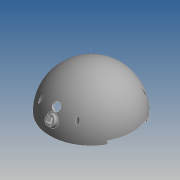
# Autodesk Inventor part: I000
Saved by Autodesk Inventor 2017 (Build 210142000, 142)
## iProperties
Created: 2018-10-05
Part Number: I000
Material: ABS
Document SubType Name: Modeling
Designer: Gilles Mottiez
Density: 1.06 g/cm^3
Appearance: Par défaut
Description: Demi-coque arrière
Mass: 97.4809 g
Surface Area: 629.597 cm^2
Volume: 91.9632 cm^3
Author: Gilles Mottiez
Autodesk Inventor part; units mm, degrees
ref_plane "YZ Plane" through (0, 0, 0) normal (1, 0, 0) x (0, 1, 0)
ref_plane "XZ Plane" through (0, 0, 0) normal (0, 1, 0) x (-1, 0, 0)
sketch "Sketch1" plane through (0, 0, 0) normal (0, 0, 1) x (1, 0, 0)
  circle A0 centre (0, 0) radius 70 construction
  line L0 (-70, 0) -> (70, 0) construction
  arc A1 (70, 0) -> (-70, 0) centre (0, 0) ccw
  line L1 (-70, 0) -> (70, 0)
  dimension "d0" = 140
  constraints: 4 end point, 4 point on circle, 2 centre point, 2 coincident, 1 collinear, 1 concentric, 1 horizontal, 1 midpoint
  measures "d0" diameter of A0
revolve "Révolution1" add sketch "Sketch1" angle 180 about axis through (-70, 0, 0) along (1, 0, 0)
sketch "Esquisse2" plane through (0, 0, 0) normal (1, 0, 0) x (0, 1, 0)
  line L0 (-70, 0) -> (70, 0) construction
  circle A0 centre (0, 0) radius 67 construction
  arc A1 (67, 0) -> (-67, 0) centre (0, 0) ccw
  line L1 (67, 0) -> (-67, 0)
  dimension "d2" = 134
  constraints: 4 point on circle, 2 centre point, 2 concentric, 2 end point, 2 point on line, 1 coincident, 1 collinear
  measures "d2" diameter of A0
revolve "Révolution2" cut sketch "Esquisse2" angle 360 about axis through (0, 67, 0) along (0, -1, 0)
sketch "Esquisse3" plane through (0, 0, 0) normal (1, 0, 0) x (0, 1, 0)
  line L0 (67, 0) -> (-67, 0) construction
  line L1 (-70, 0) -> (70, 0) construction
  arc A0 (70, 0) -> (-70, 0) centre (0, 0) ccw construction
  line L2 (32.5, 0) -> (-32.5, 0)
  line L3 (-32.5, 0) -> (-32.5, 5.5)
  line L4 (-32.5, 5.5) -> (32.5, 5.5)
  line L5 (32.5, 5.5) -> (32.5, 0)
  point P0 (0, 0)
  point P1 (0, 0)
  point P2 (0, 5.5)
  dimension "d4" = 65
  dimension "d5" = 5.5
  constraints: 8 end point, 2 midpoint, 2 parallel, 1 horizontal, 1 perpendicular, 1 point on line, 1 vertical alignment
  measures "d4" distance of L3.end L4.end
  measures "d5" distance of L4.end L2.start
extrude "Extrusion1" cut sketch "Esquisse3" along normal through all both and the other way through all
sketch "Esquisse4" plane through (0, 0, 0) normal (0, 0, -1) x (-1, 0, 0)
  line L0 (-61.998, 32.5) -> (-58.5897, 32.5) construction
  arc A0 (58.5897, 32.5) -> (-58.5897, 32.5) centre (0, 0) ccw construction
  line L1 (58.5897, 32.5) -> (61.998, 32.5) construction
  arc A1 (61.998, 32.5) -> (-61.998, 32.5) centre (0, 0) ccw construction
  arc A2 (-58.5897, -32.5) -> (58.5897, -32.5) centre (0, 0) ccw construction
  line L2 (-58.5897, -32.5) -> (-61.998, -32.5) construction
  arc A3 (-61.998, -32.5) -> (61.998, -32.5) centre (0, 0) ccw construction
  line L3 (61.998, -32.5) -> (58.5897, -32.5) construction
  arc A4 (-58.5897, -32.5) -> (58.5897, -32.5) centre (0, 0) ccw construction
  arc A5 (-58.331, 32.5) -> (-58.331, -32.5) centre (0, 0) ccw construction
  line L4 (-61.7535, 32.5) -> (-58.331, 32.5) construction
  arc A6 (-61.7535, 32.5) -> (-61.7535, -32.5) centre (0, 0) ccw construction
  line L5 (-61.7535, -32.5) -> (-58.331, -32.5) construction
  arc A7 (58.331, -32.5) -> (58.331, 32.5) centre (0, 0) ccw construction
  line L6 (58.331, -32.5) -> (61.7535, -32.5) construction
  arc A8 (61.7535, -32.5) -> (61.7535, 32.5) centre (0, 0) ccw construction
  line L7 (58.331, 32.5) -> (61.7535, 32.5) construction
  line L8 (0, 0) -> (-49.4975, 49.4975) construction
  line L9 (0, 0) -> (-69.7836, 0) construction
  circle A9 centre (0, 0) radius 63 construction
  circle A10 centre (-44.5477, 44.5477) radius 4 construction
  line L10 (-41.6309, 47.2849) -> (-44.5602, 50.0339)
  line L11 (-47.2849, 41.6309) -> (-50.2031, 44.3694)
  arc A11 (-44.5602, 50.0339) -> (-50.2031, 44.3694) centre (0, 0) ccw
  arc A12 (-47.2849, 41.6309) -> (-41.6309, 47.2849) centre (-44.5477, 44.5477) ccw
  dimension "d8" = 45
  dimension "d9" = 126
  dimension "d10" = 8
  constraints: 13 point on circle, 8 end point, 4 centre point, 2 concentric, 2 tangent, 1 coincident, 1 parallel, 1 point on line
  measures "d8" angle of L8 L9
  measures "d9" diameter of A9
  measures "d10" diameter of A10
extrude "Extrusion2" add sketch "Esquisse4" against normal up to surface
ref_plane "Plan de construction1" through (0, 0, 70) normal (0, 0, 1) x (1, 0, 0)
sketch "Esquisse6" plane through (0, 0, 70) normal (0, 0, 1) x (1, 0, 0)
  line L0 (61.998, 32.5) -> (58.5897, 32.5) construction
  arc A0 (58.5897, 32.5) -> (50.2031, 44.3694) centre (0, 0) ccw construction
  line L1 (50.2031, 44.3694) -> (47.2849, 41.6309) construction
  arc A1 (41.6309, 47.2849) -> (47.2849, 41.6309) centre (44.5477, 44.5477) ccw construction
  line L2 (41.6309, 47.2849) -> (44.5602, 50.0339) construction
  line L3 (-58.5897, 32.5) -> (-61.998, 32.5) construction
  arc A2 (61.998, 32.5) -> (-61.998, 32.5) centre (0, 0) ccw construction
  arc A3 (44.5602, 50.0339) -> (-58.5897, 32.5) centre (0, 0) ccw projected
  line L4 (58.5897, -32.5) -> (61.998, -32.5) projected
  arc A4 (-61.998, -32.5) -> (61.998, -32.5) centre (0, 0) ccw projected
  line L5 (-61.998, -32.5) -> (-58.5897, -32.5) projected
  arc A5 (-58.5897, -32.5) -> (58.5897, -32.5) centre (0, 0) ccw projected
  constraints: 1 coincident
sketch "Esquisse8" plane through (0, 0, 0) normal (0, 0, -1) x (-1, 0, 0)
  line L0 (-61.998, 32.5) -> (-58.5897, 32.5) construction
  arc A0 (-50.2031, 44.3694) -> (-58.5897, 32.5) centre (0, 0) ccw construction
  line L1 (-50.2031, 44.3694) -> (-47.2849, 41.6309) construction
  arc A1 (-47.2849, 41.6309) -> (-41.6309, 47.2849) centre (-44.5477, 44.5477) ccw construction
  line L2 (-41.6309, 47.2849) -> (-44.5602, 50.0339) construction
  line L3 (58.5897, 32.5) -> (61.998, 32.5) construction
  arc A2 (61.998, 32.5) -> (-61.998, 32.5) centre (0, 0) ccw construction
  circle A3 centre (-44.5477, 44.5477) radius 2.45
  arc A4 (58.5897, 32.5) -> (-44.5602, 50.0339) centre (0, 0) ccw projected
  line L4 (-58.5897, -32.5) -> (-61.998, -32.5) projected
  arc A5 (-61.998, -32.5) -> (61.998, -32.5) centre (0, 0) ccw projected
  line L5 (61.998, -32.5) -> (58.5897, -32.5) projected
  arc A6 (-58.5897, -32.5) -> (58.5897, -32.5) centre (0, 0) ccw projected
  dimension "d30" = 4.9
  constraints: 1 centre point, 1 coincident
  measures "d30" diameter of A3
extrude "Extrusion4" add sketch "Esquisse8" along normal blind 3 contours A3
hole "Perçage2" at (44.5477, 44.5477, 70) direction (0, 0, -1) diameter 3 end through all counterbore diameter 6 counterbore depth 65
sketch "Esquisse9" plane through (0, 0, 0) normal (0, 0, 1) x (1, 0, 0)
  arc A0 (-61.998, -32.5) -> (61.998, -32.5) centre (0, 0) ccw construction
  arc A1 (58.5897, 32.5) -> (50.2031, 44.3694) centre (0, 0) ccw construction
  arc A2 (58.5897, 32.5) -> (50.2031, 44.3694) centre (0, 0) ccw construction
  line L0 (-58.5897, -32.5) -> (-58.331, -32.5) construction
  arc A3 (-58.331, 32.5) -> (-58.331, -32.5) centre (0, 0) ccw construction
  line L1 (-58.331, 32.5) -> (-58.5897, 32.5) construction
  line L2 (44.5602, 50.0339) -> (41.6309, 47.2849) construction
  line L3 (47.2849, 41.6309) -> (50.2031, 44.3694) construction
  line L4 (58.5897, 32.5) -> (58.331, 32.5) construction
  arc A4 (58.331, -32.5) -> (58.331, 32.5) centre (0, 0) ccw construction
  line L5 (58.331, -32.5) -> (58.5897, -32.5) construction
  line L6 (50, -70) -> (-50, -70) construction
  arc A5 (-58.5897, -32.5) -> (58.5897, -32.5) centre (0, 0) ccw projected
  arc A6 (44.5602, 50.0339) -> (-58.5897, 32.5) centre (0, 0) ccw projected
  point P0 (-44.5602, -50.0339)
  point P1 (44.3694, -50.2031)
  point P2 (0, -70)
  point P3 (0, -70)
  dimension "d46" = 100
  constraints: 2 end point, 1 coincident, 1 horizontal, 1 midpoint, 1 point on circle, 1 vertical alignment, 1 other
  measures "d46" distance of L6.start L6.end
ref_plane "Plan de construction2" through (50, -70, 0) normal (0, 0.8660254, -0.5) x (-1, 0, 0)
ref_plane "Plan de construction3" through (50, -80.3923, 6) normal (0, -0.8660254, 0.5) x (1, 0, 0)
sketch "Esquisse10" plane through (50, -80.3923, 6) normal (0, -0.8660254, 0.5) x (1, 0, 0)
  line L0 (0, 0) -> (-100, 0) construction
  line L1 (-50, 0) -> (-50, 50) construction
  circle A0 centre (-50, 20) radius 7.5
  point P0 (-50, 35)
  dimension "d49" = 50
  dimension "d50" = 15
  dimension "d51" = 20
  constraints: 2 end point, 1 centre point, 1 midpoint, 1 point on line, 1 vertical
  measures "d49" distance of L1.start L1.end
  measures "d50" diameter of A0
  measures "d51" distance from line of L0 A0.centre
extrude "Extrusion5" add sketch "Esquisse10" against normal up to surface
sketch "Esquisse11" plane through (0, 0, 0) normal (0, 1, 0) x (-1, 0, 0)
  line L0 (-58.5897, 0) -> (-50.2031, 0) construction
  arc A0 (58.5897, 0) -> (58.331, 5.5) centre (0, 0) ccw construction
  line L1 (58.331, 5.5) -> (58.331, 5.5) construction
  arc A1 (58.5897, 0) -> (58.331, 5.5) centre (0, 0) ccw construction
  ellipse E0 centre (4.1003, 0) end of major axis (4.1003, -66.7315) minor radius 48.6605 (-41.6309, 22.8035) -> (-44.5602, 0) ccw construction
  ellipse E1 centre (-1.3686, 0) end of major axis (-1.3686, 66.9701) minor radius 48.8345 (-47.2849, 22.8035) -> (-50.2031, 0) ccw construction
  arc A2 (-58.331, 5.5) -> (-58.5897, 0) centre (0, 0) ccw construction
  line L2 (-58.331, 5.5) -> (-58.331, 5.5) construction
  arc A3 (-58.331, 5.5) -> (-58.5897, 0) centre (0, 0) ccw construction
  arc A4 (-61.7535, 5.5) -> (-61.998, 0) centre (0, 0) ccw construction
  line L3 (61.998, 0) -> (-61.998, 0) construction
  arc A5 (61.998, 0) -> (61.7535, 5.5) centre (0, 0) ccw construction
  line L4 (61.7535, 5.5) -> (61.7535, 5.5) construction
  arc A6 (61.998, 0) -> (61.7535, 5.5) centre (0, 0) ccw construction
  line L5 (-61.998, 0) -> (61.998, 0) construction
  arc A7 (-61.7535, 5.5) -> (-61.998, 0) centre (0, 0) ccw construction
  line L6 (-61.7535, 5.5) -> (-61.7535, 5.5) construction
  arc A8 (69.7836, 5.5) -> (-69.7836, 5.5) centre (0, 0) ccw construction
  arc A9 (66.7739, 5.5) -> (-66.7739, 5.5) centre (0, 0) ccw construction
  line L7 (0, -14) -> (0, 84) construction
  line L8 (-5, 41.2) -> (0, 41.2) construction
  line L9 (0, 47) -> (0, 67) construction
  line L10 (0, 67) -> (-5, 67) construction
  line L11 (-5, 67) -> (-5, 41.2) construction
  arc A10 (-5, 54.9909) -> (-17.6316, 64.6384) centre (-15, 54.9909) ccw
  arc A11 (0, 67) -> (-17.6316, 64.6384) centre (0, 0) ccw
  line L12 (-5, 54.9909) -> (-5, 41.2)
  line L13 (-5, 41.2) -> (-2.5, 41.2)
  line L14 (-2.5, 41.2) -> (-2.5, 51.2)
  line L15 (-2.5, 51.2) -> (0, 51.2)
  line L16 (0, 51.2) -> (0, 67)
  line L17 (-44.5602, 0) -> (58.5897, 0) projected
  line L18 (58.5897, 0) -> (-58.5897, 0) projected
  dimension "d55" = 25.8
  dimension "d56" = 10
  dimension "d57" = 10
  dimension "d58" = 5
  dimension "d59" = 10
  constraints: 18 end point, 6 point on circle, 2 centre point, 2 parallel, 2 perpendicular, 2 point on line, 2 tangent, 1 collinear, 1 concentric, 1 horizontal, 1 horizontal alignment, 1 midpoint, 1 vertical, 4 other
  measures "d55" distance from line of L9.end L8
  measures "d56" distance between parallel lines of L8 L15
  measures "d57" diameter of L12 L16
  measures "d58" diameter of L14 L16
  measures "d59" radius of A10
revolve "Révolution3" add sketch "Esquisse11" angle 360 about axis through (0, 0, 51.2) along (0, 0, 1)
mirror "Symétrie1" about plane through (0, 0, 0) normal (1, 0, 0) of "Extrusion2", "Extrusion4", "Perçage2"
sketch "Esquisse12" plane through (0, 0, 0) normal (0, 0, -1) x (-1, 0, 0)
  line L0 (-58.5897, -32.5) -> (-61.998, -32.5) construction
  arc A0 (-61.998, -32.5) -> (61.998, -32.5) centre (0, 0) ccw construction
  line L1 (61.998, -32.5) -> (58.5897, -32.5) construction
  arc A1 (-58.5897, -32.5) -> (58.5897, -32.5) centre (0, 0) ccw construction
  line L2 (0, 0) -> (-33.5, -58.0237) construction
  arc A2 (-58.331, 32.5) -> (-58.331, -32.5) centre (0, 0) ccw construction
  line L3 (-61.7535, 32.5) -> (-58.331, 32.5) construction
  arc A3 (-61.7535, 32.5) -> (-61.7535, -32.5) centre (0, 0) ccw construction
  line L4 (-61.7535, -32.5) -> (-58.331, -32.5) construction
  line L5 (0, 0) -> (-66.7739, 0) construction
  circle A4 centre (0, 0) radius 63 construction
  circle A5 centre (-31.5, -54.5596) radius 4 construction
  line L6 (-34.8989, -52.4506) -> (-37.0088, -55.8511)
  line L7 (-27.9742, -56.4486) -> (-29.8641, -59.9761)
  arc A6 (-27.9742, -56.4486) -> (-34.8989, -52.4506) centre (-31.5, -54.5596) ccw
  arc A7 (-37.0088, -55.8511) -> (-29.8641, -59.9761) centre (0, 0) ccw
  dimension "d61" = 60
  dimension "d62" = 126
  dimension "d63" = 8
  constraints: 13 point on circle, 8 end point, 4 centre point, 4 tangent, 1 coincident, 1 horizontal, 1 point on line
  measures "d61" angle of L2 L5
  measures "d62" diameter of A4
  measures "d63" diameter of A5
extrude "Extrusion6" add sketch "Esquisse12" against normal up to next
sketch "Esquisse13" plane through (0, 0, 0) normal (0, 0, -1) x (-1, 0, 0)
  line L0 (-34.8989, -52.4506) -> (-37.0088, -55.8511) construction
  arc A0 (-58.5897, -32.5) -> (-37.0088, -55.8511) centre (0, 0) ccw construction
  line L1 (-58.5897, -32.5) -> (-61.998, -32.5) construction
  arc A1 (-61.998, -32.5) -> (61.998, -32.5) centre (0, 0) ccw construction
  line L2 (61.998, -32.5) -> (58.5897, -32.5) construction
  arc A2 (-29.8641, -59.9761) -> (58.5897, -32.5) centre (0, 0) ccw construction
  line L3 (-29.8641, -59.9761) -> (-27.9742, -56.4486) construction
  arc A3 (-27.9742, -56.4486) -> (-34.8989, -52.4506) centre (-31.5, -54.5596) ccw construction
  circle A4 centre (-31.5, -54.5596) radius 2.45
  dimension "d66" = 4.9
  constraints: 1 centre point, 1 coincident
  measures "d66" diameter of A4
extrude "Extrusion7" add sketch "Esquisse13" along normal blind 3
sketch "Esquisse15" plane through (0, 0, 70) normal (0, 0, 1) x (1, 0, 0)
  circle A0 centre (31.5, -54.5596) radius 2.45 construction
  point P0 (0, 0)
  constraints: 1 coincident
hole "Perçage3" at (31.5, -54.5596, 70) direction (0, 0, -1) diameter 3 end through all counterbore diameter 5 counterbore depth 65
mirror "Symétrie2" about plane through (0, 0, 0) normal (1, 0, 0) of "Extrusion7", "Perçage3", "Extrusion6"
fillet "Congé1" radius 3 1 edges at (-7.5, -66.3594, 20.9803)
fillet "Congé2" radius 1 4 edges at (61.9368, 32.5, 2.7527) (61.9368, -32.5, 2.7527) (-61.9368, -32.5, 2.7527) (-61.9368, 32.5, 2.7527)
sketch "Esquisse16" plane through (50, -80.3923, 6) normal (0, -0.8660254, 0.5) x (1, 0, 0)
  ellipse E0 centre (-50, 51.9928) end of major axis (-111.1963, 51.9928) minor radius 52.9975 (-110.9486, 56.7559) -> (-111.1963, 51.9928) ccw construction
  ellipse E1 centre (-50, 39.7631) end of major axis (-119.7836, 39.7631) minor radius 34.8918 (-110.9486, 56.7559) -> (-110.9486, 22.7704) ccw construction
  ellipse E2 centre (-50, 18.0072) end of major axis (-111.1963, 18.0072) minor radius 52.9975 (-110.9486, 22.7704) -> (-111.1963, 18.0072) ccw construction
  ellipse E3 centre (-50, 35) end of major axis (-120, 35) minor radius 35 (-111.1963, 18.0072) -> (11.1963, 18.0072) ccw construction
  ellipse E4 centre (-50, 18.0072) end of major axis (11.1963, 18.0072) minor radius 52.9975 (11.1963, 18.0072) -> (10.9486, 22.7704) ccw construction
  ellipse E5 centre (-50, 39.7631) end of major axis (-119.7836, 39.7631) minor radius 34.8918 (10.9486, 22.7704) -> (10.9486, 56.7559) ccw construction
  ellipse E6 centre (-50, 51.9928) end of major axis (11.1963, 51.9928) minor radius 52.9975 (11.1963, 51.9928) -> (10.9486, 56.7559) ccw construction
  ellipse E7 centre (-50, 35) end of major axis (-120, 35) minor radius 35 (11.1963, 51.9928) -> (-111.1963, 51.9928) ccw construction
  line L0 (-50, 51.9928) -> (-50, 18.0072) construction
  circle A0 centre (-50, 38.0072) radius 6
  point P0 (-50, 35)
  dimension "d78" = 12
  dimension "d79" = 20
  constraints: 2 end point, 1 centre point, 1 point on line, 1 vertical, 13 other
  measures "d78" diameter of A0
  measures "d79" distance of point (-50, 18.007) A0.centre
extrude "Extrusion8" cut sketch "Esquisse16" against normal through all
sketch "Esquisse17" plane through (50, -80.3923, 6) normal (0, -0.8660254, 0.5) x (1, 0, 0)
  arc A0 (-53.4279, 26.6708) -> (-46.5721, 26.6708) centre (-50, 20) ccw construction
  line L0 (-54, 16) -> (-46, 16)
  line L1 (-46, 16) -> (-46, 24)
  line L2 (-46, 24) -> (-54, 24)
  line L3 (-54, 24) -> (-54, 16)
  line L4 (-54, 16) -> (-46, 24) construction
  line L5 (-46, 16) -> (-54, 24) construction
  point P0 (-50, 35)
  dimension "d82" = 8
  dimension "d83" = 8
  constraints: 12 end point, 2 midpoint, 2 parallel, 1 horizontal, 1 horizontal alignment, 1 perpendicular
  measures "d82" distance of L2.end L1.end
  measures "d83" distance of L1.end L0.end
extrude "Extrusion9" cut sketch "Esquisse17" against normal blind 11
fillet "Congé3" radius 0.5 2 edges at (-6, -56.2283, 35.9357) (-6, -58.8387, 37.4433)
